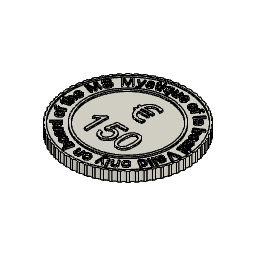
birthday_chip (Autodesk Fusion 360 design; units mm, degrees)
Autodesk Fusion 360 part; units mm, degrees
(part 1 of 2)
sketch "Skizze1" plane through (0, 0, 0) normal (0, 0, 1) x (1, 0, 0)
  circle A0 centre (0, 0) radius 25
  circle A1 centre (0, 0) radius 23.6538
  dimension "d1" = 50
  dimension "d4" = -1.3462
  constraint coincident A0.centre A1.centre
  measures "d1" diameter of A0
extrude "Extrusion1" add sketch "Skizze1" along normal blind 4 contours A0 | A1
sketch "Skizze2" plane through (0, 0, 4) normal (0, 0, 1) x (-1, 0, 0)
  circle A0 centre (0, 0) radius 25
  circle A1 centre (0, 0) radius 24.1386
  dimension "d5" = -0.8614
extrude "Extrusion2" cut sketch "Skizze2" against normal blind 0.6 contours A1
sketch "Skizze3" plane through (0, 0, 3.4) normal (0, 0, 1) x (-1, 0, 0)
  circle A0 centre (0, 0) radius 24.1386
  circle A1 centre (0, 0) radius 17.6628
  circle A2 centre (0, 0) radius 16.7912
  dimension "d8" = -6.4758
  dimension "d9" = -7.3474
extrude "Extrusion3" add sketch "Skizze3" along normal blind 0.6 contours A1
sketch "Skizze4" plane through (0, 0, 3.4) normal (0, 0, 1) x (-1, 0, 0)
  circle A0 centre (0, 0) radius 16.7912
  spline S0 degree 2 poles (-0.7975, -6.5191) (-0.2245, -6.5191) (0.1643, -6.2428) knots 0 0 0 1 1 1
  spline S1 degree 2 poles (0.1643, -6.2428) (0.3962, -6.0791) (0.5838, -5.779) knots 0 0 0 1 1 1
  spline S2 degree 2 poles (0.5838, -5.779) (0.7748, -5.4686) (0.8089, -5.1889) knots 0 0 0 1 1 1
  line L0 (0.8089, -5.1889) -> (-1.5172, -5.1889)
  line L1 (-1.5172, -5.1889) -> (-1.4251, -4.7319)
  line L2 (-1.4251, -4.7319) -> (0.8634, -4.7319)
  spline S3 degree 2 poles (0.8634, -4.7319) (0.8669, -4.6603) (0.8669, -4.5955) knots 0 0 0 1 1 1
  spline S4 degree 2 poles (0.8669, -4.5955) (0.8669, -4.3329) (0.8634, -4.2817) knots 0 0 0 1 1 1
  line L3 (0.8634, -4.2817) -> (-1.333, -4.2817)
  line L4 (-1.333, -4.2817) -> (-1.2375, -3.8247)
  line L5 (-1.2375, -3.8247) -> (0.7918, -3.8247)
  spline S5 degree 2 poles (0.7918, -3.8247) (0.6486, -3.0437) (0.1029, -2.7162) knots 0 0 0 1 1 1
  spline S6 degree 2 poles (0.1029, -2.7162) (-0.2894, -2.4809) (-0.7464, -2.4809) knots 0 0 0 1 1 1
  spline S7 degree 2 poles (-0.7464, -2.4809) (-1.3842, -2.4809) (-1.7423, -2.8151) knots 0 0 0 1 1 1
  line L6 (-1.7423, -2.8151) -> (-1.7423, -2.1126)
  spline S8 degree 2 poles (-1.7423, -2.1126) (-1.316, -1.9147) (-0.8009, -1.9147) knots 0 0 0 1 1 1
  spline S9 degree 2 poles (-0.8009, -1.9147) (0.7407, -1.9147) (1.283, -3.1971) knots 0 0 0 1 1 1
  spline S10 degree 2 poles (1.283, -3.1971) (1.3921, -3.4563) (1.4705, -3.8247) knots 0 0 0 1 1 1
  line L7 (1.4705, -3.8247) -> (1.9924, -3.8247)
  line L8 (1.9924, -3.8247) -> (1.8969, -4.2817)
  line L9 (1.8969, -4.2817) -> (1.5388, -4.2817)
  spline S11 degree 2 poles (1.5388, -4.2817) (1.549, -4.425) (1.549, -4.5921) knots 0 0 0 1 1 1
  spline S12 degree 2 poles (1.549, -4.5921) (1.549, -4.6603) (1.5456, -4.7319) knots 0 0 0 1 1 1
  line L10 (1.5456, -4.7319) -> (1.9924, -4.7319)
  line L11 (1.9924, -4.7319) -> (1.8969, -5.1889)
  line L12 (1.8969, -5.1889) -> (1.5012, -5.1889)
  spline S13 degree 2 poles (1.5012, -5.1889) (1.2898, -6.3008) (0.3996, -6.7851) knots 0 0 0 1 1 1
  spline S14 degree 2 poles (0.3996, -6.7851) (-0.1495, -7.0853) (-0.8112, -7.0853) knots 0 0 0 1 1 1
  spline S15 degree 2 poles (-0.8112, -7.0853) (-1.4456, -7.0853) (-1.8787, -6.809) knots 0 0 0 1 1 1
  line L13 (-1.8787, -6.809) -> (-1.7423, -6.1746)
  spline S16 degree 2 poles (-1.7423, -6.1746) (-1.3262, -6.5191) (-0.7975, -6.5191) knots 0 0 0 1 1 1
  line L14 (3.1793, 5.8035) -> (3.7932, 5.8035)
  line L15 (3.7932, 5.8035) -> (3.7932, 1.8915)
  spline S17 degree 2 poles (3.7932, 1.8915) (4.0149, 2.103) (4.3747, 2.3145) knots 0 0 0 1 1 1
  spline S18 degree 2 poles (4.3747, 2.3145) (4.7345, 2.5259) (5.021, 2.6316) knots 0 0 0 1 1 1
  line L16 (5.021, 2.6316) -> (5.021, 2.0382)
  spline S19 degree 2 poles (5.021, 2.0382) (4.506, 1.796) (4.1206, 1.4516) knots 0 0 0 1 1 1
  spline S20 degree 2 poles (4.1206, 1.4516) (3.7352, 1.1071) (3.5749, 0.7831) knots 0 0 0 1 1 1
  line L17 (3.5749, 0.7831) -> (3.1793, 0.7831)
  line L18 (3.1793, 0.7831) -> (3.1793, 5.8035)
  line L19 (1.607, 4.4939) -> (0.9624, 4.4393)
  spline S21 degree 2 poles (0.9624, 4.4393) (0.8907, 4.91) (0.6298, 5.147) knots 0 0 0 1 1 1
  spline S22 degree 2 poles (0.6298, 5.147) (0.3689, 5.384) (0.0006, 5.384) knots 0 0 0 1 1 1
  spline S23 degree 2 poles (0.0006, 5.384) (-0.4428, 5.384) (-0.7498, 5.0498) knots 0 0 0 1 1 1
  spline S24 degree 2 poles (-0.7498, 5.0498) (-1.0567, 4.7156) (-1.0567, 4.163) knots 0 0 0 1 1 1
  spline S25 degree 2 poles (-1.0567, 4.163) (-1.0567, 3.6378) (-0.7617, 3.3342) knots 0 0 0 1 1 1
  spline S26 degree 2 poles (-0.7617, 3.3342) (-0.4667, 3.0307) (0.0108, 3.0307) knots 0 0 0 1 1 1
  spline S27 degree 2 poles (0.0108, 3.0307) (0.3075, 3.0307) (0.5463, 3.1654) knots 0 0 0 1 1 1
  spline S28 degree 2 poles (0.5463, 3.1654) (0.785, 3.3001) (0.9214, 3.515) knots 0 0 0 1 1 1
  line L20 (0.9214, 3.515) -> (1.4978, 3.44)
  line L21 (1.4978, 3.44) -> (1.0135, 0.8718)
  line L22 (1.0135, 0.8718) -> (-1.4728, 0.8718)
  line L23 (-1.4728, 0.8718) -> (-1.4728, 1.4584)
  line L24 (-1.4728, 1.4584) -> (0.5224, 1.4584)
  line L25 (0.5224, 1.4584) -> (0.7918, 2.8022)
  spline S29 degree 2 poles (0.7918, 2.8022) (0.3416, 2.4884) (-0.1529, 2.4884) knots 0 0 0 1 1 1
  spline S30 degree 2 poles (-0.1529, 2.4884) (-0.8078, 2.4884) (-1.258, 2.942) knots 0 0 0 1 1 1
  spline S31 degree 2 poles (-1.258, 2.942) (-1.7082, 3.3956) (-1.7082, 4.1085) knots 0 0 0 1 1 1
  spline S32 degree 2 poles (-1.7082, 4.1085) (-1.7082, 4.7872) (-1.3125, 5.2817) knots 0 0 0 1 1 1
  spline S33 degree 2 poles (-1.3125, 5.2817) (-0.8316, 5.8888) (0.0006, 5.8888) knots 0 0 0 1 1 1
  spline S34 degree 2 poles (0.0006, 5.8888) (0.6827, 5.8888) (1.1141, 5.5068) knots 0 0 0 1 1 1
  spline S35 degree 2 poles (1.1141, 5.5068) (1.5456, 5.1248) (1.607, 4.4939) knots 0 0 0 1 1 1
  spline S36 degree 2 poles (-2.2778, 3.3377) (-2.2778, 2.4509) (-2.4602, 1.9103) knots 0 0 0 1 1 1
  spline S37 degree 2 poles (-2.4602, 1.9103) (-2.6427, 1.3697) (-3.0025, 1.0764) knots 0 0 0 1 1 1
  spline S38 degree 2 poles (-3.0025, 1.0764) (-3.3623, 0.7831) (-3.908, 0.7831) knots 0 0 0 1 1 1
  spline S39 degree 2 poles (-3.908, 0.7831) (-4.3105, 0.7831) (-4.614, 0.9451) knots 0 0 0 1 1 1
  spline S40 degree 2 poles (-4.614, 0.9451) (-4.9176, 1.1071) (-5.1154, 1.4123) knots 0 0 0 1 1 1
  spline S41 degree 2 poles (-5.1154, 1.4123) (-5.3132, 1.7176) (-5.4258, 2.1559) knots 0 0 0 1 1 1
  spline S42 degree 2 poles (-5.4258, 2.1559) (-5.5383, 2.5941) (-5.5383, 3.3377) knots 0 0 0 1 1 1
  spline S43 degree 2 poles (-5.5383, 3.3377) (-5.5383, 4.2176) (-5.3576, 4.7582) knots 0 0 0 1 1 1
  spline S44 degree 2 poles (-5.3576, 4.7582) (-5.1768, 5.2988) (-4.817, 5.5938) knots 0 0 0 1 1 1
  spline S45 degree 2 poles (-4.817, 5.5938) (-4.4572, 5.8888) (-3.908, 5.8888) knots 0 0 0 1 1 1
  spline S46 degree 2 poles (-3.908, 5.8888) (-3.185, 5.8888) (-2.7723, 5.3704) knots 0 0 0 1 1 1
  spline S47 degree 2 poles (-2.7723, 5.3704) (-2.2778, 4.7462) (-2.2778, 3.3377) knots 0 0 0 1 1 1
  spline S48 degree 2 poles (-2.9087, 3.3377) (-2.9087, 4.5689) (-3.1969, 4.9765) knots 0 0 0 1 1 1
  spline S49 degree 2 poles (-3.1969, 4.9765) (-3.4851, 5.384) (-3.908, 5.384) knots 0 0 0 1 1 1
  spline S50 degree 2 poles (-3.908, 5.384) (-4.331, 5.384) (-4.6192, 4.9748) knots 0 0 0 1 1 1
  spline S51 degree 2 poles (-4.6192, 4.9748) (-4.9074, 4.5655) (-4.9074, 3.3377) knots 0 0 0 1 1 1
  spline S52 degree 2 poles (-4.9074, 3.3377) (-4.9074, 2.103) (-4.6192, 1.6971) knots 0 0 0 1 1 1
  spline S53 degree 2 poles (-4.6192, 1.6971) (-4.331, 1.2913) (-3.9012, 1.2913) knots 0 0 0 1 1 1
  spline S54 degree 2 poles (-3.9012, 1.2913) (-3.4783, 1.2913) (-3.2259, 1.6494) knots 0 0 0 1 1 1
  spline S55 degree 2 poles (-3.2259, 1.6494) (-2.9087, 2.1064) (-2.9087, 3.3377) knots 0 0 0 1 1 1
sketch "Skizze5" plane through (0, 0, 3.4) normal (0, 0, 1) x (-1, 0, 0)
  circle A0 centre (0, 0) radius 16.7912
  spline S0 degree 2 poles (-0.97, -11.1344) (0.0614, -11.1344) (0.7613, -10.6371) knots 0 0 0 1 1 1
  spline S1 degree 2 poles (0.7613, -10.6371) (1.1787, -10.3424) (1.5164, -9.8022) knots 0 0 0 1 1 1
  spline S2 degree 2 poles (1.5164, -9.8022) (1.8602, -9.2435) (1.9216, -8.7401) knots 0 0 0 1 1 1
  line L0 (1.9216, -8.7401) -> (-2.2653, -8.7401)
  line L1 (-2.2653, -8.7401) -> (-2.0996, -7.9175)
  line L2 (-2.0996, -7.9175) -> (2.0198, -7.9175)
  spline S3 degree 2 poles (2.0198, -7.9175) (2.0259, -7.7885) (2.0259, -7.6719) knots 0 0 0 1 1 1
  spline S4 degree 2 poles (2.0259, -7.6719) (2.0259, -7.1992) (2.0198, -7.1071) knots 0 0 0 1 1 1
  line L3 (2.0198, -7.1071) -> (-1.9338, -7.1071)
  line L4 (-1.9338, -7.1071) -> (-1.7619, -6.2844)
  line L5 (-1.7619, -6.2844) -> (1.8909, -6.2844)
  spline S5 degree 2 poles (1.8909, -6.2844) (1.633, -4.8786) (0.6508, -4.2892) knots 0 0 0 1 1 1
  spline S6 degree 2 poles (0.6508, -4.2892) (-0.0553, -3.8656) (-0.8779, -3.8656) knots 0 0 0 1 1 1
  spline S7 degree 2 poles (-0.8779, -3.8656) (-2.0259, -3.8656) (-2.6705, -4.4673) knots 0 0 0 1 1 1
  line L6 (-2.6705, -4.4673) -> (-2.6705, -3.2026)
  spline S8 degree 2 poles (-2.6705, -3.2026) (-1.9031, -2.8465) (-0.9761, -2.8465) knots 0 0 0 1 1 1
  spline S9 degree 2 poles (-0.9761, -2.8465) (1.7988, -2.8465) (2.7749, -5.1548) knots 0 0 0 1 1 1
  spline S10 degree 2 poles (2.7749, -5.1548) (2.9714, -5.6214) (3.1126, -6.2844) knots 0 0 0 1 1 1
  line L7 (3.1126, -6.2844) -> (4.0518, -6.2844)
  line L8 (4.0518, -6.2844) -> (3.8799, -7.1071)
  line L9 (3.8799, -7.1071) -> (3.2353, -7.1071)
  spline S11 degree 2 poles (3.2353, -7.1071) (3.2538, -7.3649) (3.2538, -7.6658) knots 0 0 0 1 1 1
  spline S12 degree 2 poles (3.2538, -7.6658) (3.2538, -7.7885) (3.2476, -7.9175) knots 0 0 0 1 1 1
  line L10 (3.2476, -7.9175) -> (4.0518, -7.9175)
  line L11 (4.0518, -7.9175) -> (3.8799, -8.7401)
  line L12 (3.8799, -8.7401) -> (3.1678, -8.7401)
  spline S13 degree 2 poles (3.1678, -8.7401) (2.7872, -10.7415) (1.1849, -11.6132) knots 0 0 0 1 1 1
  spline S14 degree 2 poles (1.1849, -11.6132) (0.1965, -12.1535) (-0.9945, -12.1535) knots 0 0 0 1 1 1
  spline S15 degree 2 poles (-0.9945, -12.1535) (-2.1364, -12.1535) (-2.9161, -11.6562) knots 0 0 0 1 1 1
  line L13 (-2.9161, -11.6562) -> (-2.6705, -10.5143)
  spline S16 degree 2 poles (-2.6705, -10.5143) (-1.9216, -11.1344) (-0.97, -11.1344) knots 0 0 0 1 1 1
  line L14 (6.1883, 11.0464) -> (7.2933, 11.0464)
  line L15 (7.2933, 11.0464) -> (7.2933, 4.0048)
  spline S17 degree 2 poles (7.2933, 4.0048) (7.6924, 4.3854) (8.34, 4.766) knots 0 0 0 1 1 1
  spline S18 degree 2 poles (8.34, 4.766) (8.9877, 5.1467) (9.5034, 5.337) knots 0 0 0 1 1 1
  line L16 (9.5034, 5.337) -> (9.5034, 4.2688)
  spline S19 degree 2 poles (9.5034, 4.2688) (8.5764, 3.8329) (7.8827, 3.2128) knots 0 0 0 1 1 1
  spline S20 degree 2 poles (7.8827, 3.2128) (7.1889, 2.5928) (6.9004, 2.0096) knots 0 0 0 1 1 1
  line L17 (6.9004, 2.0096) -> (6.1883, 2.0096)
  line L18 (6.1883, 2.0096) -> (6.1883, 11.0464)
  line L19 (3.3581, 8.6889) -> (2.1978, 8.5907)
  spline S21 degree 2 poles (2.1978, 8.5907) (2.0689, 9.4379) (1.5992, 9.8646) knots 0 0 0 1 1 1
  spline S22 degree 2 poles (1.5992, 9.8646) (1.1296, 10.2913) (0.4666, 10.2913) knots 0 0 0 1 1 1
  spline S23 degree 2 poles (0.4666, 10.2913) (-0.3315, 10.2913) (-0.884, 9.6896) knots 0 0 0 1 1 1
  spline S24 degree 2 poles (-0.884, 9.6896) (-1.4366, 9.088) (-1.4366, 8.0935) knots 0 0 0 1 1 1
  spline S25 degree 2 poles (-1.4366, 8.0935) (-1.4366, 7.148) (-0.9055, 6.6016) knots 0 0 0 1 1 1
  spline S26 degree 2 poles (-0.9055, 6.6016) (-0.3745, 6.0553) (0.485, 6.0553) knots 0 0 0 1 1 1
  spline S27 degree 2 poles (0.485, 6.0553) (1.0191, 6.0553) (1.4488, 6.2977) knots 0 0 0 1 1 1
  spline S28 degree 2 poles (1.4488, 6.2977) (1.8786, 6.5402) (2.1241, 6.927) knots 0 0 0 1 1 1
  line L20 (2.1241, 6.927) -> (3.1617, 6.792)
  line L21 (3.1617, 6.792) -> (2.2899, 2.1692)
  line L22 (2.2899, 2.1692) -> (-2.1855, 2.1692)
  line L23 (-2.1855, 2.1692) -> (-2.1855, 3.2251)
  line L24 (-2.1855, 3.2251) -> (1.4059, 3.2251)
  line L25 (1.4059, 3.2251) -> (1.8909, 5.6439)
  spline S29 degree 2 poles (1.8909, 5.6439) (1.0805, 5.0791) (0.1903, 5.0791) knots 0 0 0 1 1 1
  spline S30 degree 2 poles (0.1903, 5.0791) (-0.9884, 5.0791) (-1.7988, 5.8956) knots 0 0 0 1 1 1
  spline S31 degree 2 poles (-1.7988, 5.8956) (-2.6091, 6.7121) (-2.6091, 7.9952) knots 0 0 0 1 1 1
  spline S32 degree 2 poles (-2.6091, 7.9952) (-2.6091, 9.2169) (-1.897, 10.1071) knots 0 0 0 1 1 1
  spline S33 degree 2 poles (-1.897, 10.1071) (-1.0314, 11.1999) (0.4666, 11.1999) knots 0 0 0 1 1 1
  spline S34 degree 2 poles (0.4666, 11.1999) (1.6944, 11.1999) (2.471, 10.5123) knots 0 0 0 1 1 1
  spline S35 degree 2 poles (2.471, 10.5123) (3.2476, 9.8247) (3.3581, 8.6889) knots 0 0 0 1 1 1
  spline S36 degree 2 poles (-3.6344, 6.6078) (-3.6344, 5.0116) (-3.9628, 4.0385) knots 0 0 0 1 1 1
  spline S37 degree 2 poles (-3.9628, 4.0385) (-4.2913, 3.0655) (-4.9389, 2.5375) knots 0 0 0 1 1 1
  spline S38 degree 2 poles (-4.9389, 2.5375) (-5.5866, 2.0096) (-6.5689, 2.0096) knots 0 0 0 1 1 1
  spline S39 degree 2 poles (-6.5689, 2.0096) (-7.2933, 2.0096) (-7.8397, 2.3012) knots 0 0 0 1 1 1
  spline S40 degree 2 poles (-7.8397, 2.3012) (-8.3861, 2.5928) (-8.7422, 3.1422) knots 0 0 0 1 1 1
  spline S41 degree 2 poles (-8.7422, 3.1422) (-9.0982, 3.6917) (-9.3008, 4.4806) knots 0 0 0 1 1 1
  spline S42 degree 2 poles (-9.3008, 4.4806) (-9.5034, 5.2694) (-9.5034, 6.6078) knots 0 0 0 1 1 1
  spline S43 degree 2 poles (-9.5034, 6.6078) (-9.5034, 8.1917) (-9.178, 9.1647) knots 0 0 0 1 1 1
  spline S44 degree 2 poles (-9.178, 9.1647) (-8.8527, 10.1378) (-8.205, 10.6688) knots 0 0 0 1 1 1
  spline S45 degree 2 poles (-8.205, 10.6688) (-7.5573, 11.1999) (-6.5689, 11.1999) knots 0 0 0 1 1 1
  spline S46 degree 2 poles (-6.5689, 11.1999) (-5.2674, 11.1999) (-4.5246, 10.2667) knots 0 0 0 1 1 1
  spline S47 degree 2 poles (-4.5246, 10.2667) (-3.6344, 9.1432) (-3.6344, 6.6078) knots 0 0 0 1 1 1
  spline S48 degree 2 poles (-4.7701, 6.6078) (-4.7701, 8.824) (-5.2889, 9.5576) knots 0 0 0 1 1 1
  spline S49 degree 2 poles (-5.2889, 9.5576) (-5.8076, 10.2913) (-6.5689, 10.2913) knots 0 0 0 1 1 1
  spline S50 degree 2 poles (-6.5689, 10.2913) (-7.3301, 10.2913) (-7.8489, 9.5546) knots 0 0 0 1 1 1
  spline S51 degree 2 poles (-7.8489, 9.5546) (-8.3677, 8.8179) (-8.3677, 6.6078) knots 0 0 0 1 1 1
  spline S52 degree 2 poles (-8.3677, 6.6078) (-8.3677, 4.3854) (-7.8489, 3.6548) knots 0 0 0 1 1 1
  spline S53 degree 2 poles (-7.8489, 3.6548) (-7.3301, 2.9243) (-6.5566, 2.9243) knots 0 0 0 1 1 1
  spline S54 degree 2 poles (-6.5566, 2.9243) (-5.7954, 2.9243) (-5.3411, 3.5689) knots 0 0 0 1 1 1
  spline S55 degree 2 poles (-5.3411, 3.5689) (-4.7701, 4.3915) (-4.7701, 6.6078) knots 0 0 0 1 1 1
extrude "Extrusion5" add sketch "Skizze5" along normal blind 0.6 contours S0 S1 S2 L0 L1 L2 S3 S4 L3 L4 L5 S5 S6 S7 L6 S8 S9 S10 L7 L8 L9 S11 S12 L10 L11 L12 S13 S14 S15 L13 S16 | L14 L15 S17 S18 L16 S19 S20 L17 L18 | L19 S21 S22 S23 S24 S25 S26 S27 S28 L20 L21 L22 L23 L24 L25 S29 S30 S31 S32 S33 S34 S35 | S36 S37 S38 S39 S40 S41 S42 S43 S44 S45 S46 S47
sketch "Skizze7" plane through (0, 0, 4) normal (0, 0, 1) x (-1, 0, 0)
  circle A0 centre (0, 0) radius 24.1386
  circle A1 centre (0, 0) radius 25
  circle A2 centre (0, -26) radius 1.329
  circle A3 centre (2.7177, -25.8576) radius 1.329
  circle A4 centre (5.4057, -25.4318) radius 1.329
  circle A5 centre (8.0344, -24.7275) radius 1.329
  circle A6 centre (10.5752, -23.7522) radius 1.329
  circle A7 centre (13, -22.5167) radius 1.329
  circle A8 centre (15.2824, -21.0344) radius 1.329
  circle A9 centre (17.3974, -19.3218) radius 1.329
  circle A10 centre (19.3218, -17.3974) radius 1.329
  circle A11 centre (21.0344, -15.2824) radius 1.329
  circle A12 centre (22.5167, -13) radius 1.329
  circle A13 centre (23.7522, -10.5752) radius 1.329
  circle A14 centre (24.7275, -8.0344) radius 1.329
  circle A15 centre (25.4318, -5.4057) radius 1.329
  circle A16 centre (25.8576, -2.7177) radius 1.329
  circle A17 centre (26, 0) radius 1.329
  circle A18 centre (25.8576, 2.7177) radius 1.329
  circle A19 centre (25.4318, 5.4057) radius 1.329
  circle A20 centre (24.7275, 8.0344) radius 1.329
  circle A21 centre (23.7522, 10.5752) radius 1.329
  circle A22 centre (22.5167, 13) radius 1.329
  circle A23 centre (21.0344, 15.2824) radius 1.329
  circle A24 centre (19.3218, 17.3974) radius 1.329
  circle A25 centre (17.3974, 19.3218) radius 1.329
  circle A26 centre (15.2824, 21.0344) radius 1.329
  circle A27 centre (13, 22.5167) radius 1.329
  circle A28 centre (10.5752, 23.7522) radius 1.329
  circle A29 centre (8.0344, 24.7275) radius 1.329
  circle A30 centre (5.4057, 25.4318) radius 1.329
  circle A31 centre (2.7177, 25.8576) radius 1.329
  circle A32 centre (0, 26) radius 1.329
  circle A33 centre (-2.7177, 25.8576) radius 1.329
  circle A34 centre (-5.4057, 25.4318) radius 1.329
  circle A35 centre (-8.0344, 24.7275) radius 1.329
  circle A36 centre (-10.5752, 23.7522) radius 1.329
  circle A37 centre (-13, 22.5167) radius 1.329
  circle A38 centre (-15.2824, 21.0344) radius 1.329
  circle A39 centre (-17.3974, 19.3218) radius 1.329
  circle A40 centre (-19.3218, 17.3974) radius 1.329
  circle A41 centre (-21.0344, 15.2824) radius 1.329
  circle A42 centre (-22.5167, 13) radius 1.329
  circle A43 centre (-23.7522, 10.5752) radius 1.329
  circle A44 centre (-24.7275, 8.0344) radius 1.329
  circle A45 centre (-25.4318, 5.4057) radius 1.329
  circle A46 centre (-25.8576, 2.7177) radius 1.329
  circle A47 centre (-26, 0) radius 1.329
  circle A48 centre (-25.8576, -2.7177) radius 1.329
  circle A49 centre (-25.4318, -5.4057) radius 1.329
  circle A50 centre (-24.7275, -8.0344) radius 1.329
  circle A51 centre (-23.7522, -10.5752) radius 1.329
  circle A52 centre (-22.5167, -13) radius 1.329
  circle A53 centre (-21.0344, -15.2824) radius 1.329
  circle A54 centre (-19.3218, -17.3974) radius 1.329
  circle A55 centre (-17.3974, -19.3218) radius 1.329
  circle A56 centre (-15.2824, -21.0344) radius 1.329
  circle A57 centre (-13, -22.5167) radius 1.329
  circle A58 centre (-10.5752, -23.7522) radius 1.329
  circle A59 centre (-8.0344, -24.7275) radius 1.329
  circle A60 centre (-5.4057, -25.4318) radius 1.329
  circle A61 centre (-2.7177, -25.8576) radius 1.329
  dimension "d22" = 2.6579
  dimension "d24" = 360
  measures "d22" diameter of A2
extrude "Extrusion7" cut sketch "Skizze7" against normal blind 10 contours A1 A17 | A1 A18 | A1 A16 | A1 A19 | A1 A15 | A1 A20 | A1 A14 | A1 A21 | A1 A13 | A1 A22 | A1 A12 | A1 A23 | A1 A11 | A1 A24 | A1 A10 | A1 A25 | A1 A9 | A1 A26 | A1 A8 | A1 A27 | A1 A7 | A1 A28 | A1 A6 | A1 A29 | A1 A5 | A1 A30 | A1 A4 | A1 A31 | A1 A3 | A1 A32 | A1 A2 | A1 A33 | A1 A61 | A1 A34 | A1 A60 | A1 A35 | A1 A59 | A1 A36 | A1 A58 | A1 A37 | A1 A57 | A1 A38 | A1 A56 | A1 A39 | A1 A55 | A1 A40 | A1 A54 | A1 A41 | A1 A53 | A1 A42 | A1 A52 | A1 A43 | A1 A51 | A1 A44 | A1 A50 | A1 A45 | A1 A49 | A1 A46 | A1 A48 | A1 A47 picked at (24.8942, -0.1574) picked at (24.7529, 2.6016) picked at (24.7529, -2.6016) picked at (24.3454, 5.1748) picked at (24.3454, -5.1748) picked at (23.6711, 7.6912) picked at (23.6711, -7.6912) picked at (22.7375, 10.1234) picked at (22.7375, -10.1234) picked at (21.5547, 12.4446) picked at (21.5547, -12.4446) picked at (20.1358, 14.6295) picked at (20.1358, -14.6295) picked at (18.4963, 16.6542) picked at (18.4963, -16.6542) picked at (16.6542, 18.4963) picked at (16.6542, -18.4963) picked at (14.6295, 20.1358) picked at (14.6295, -20.1358) picked at (12.4446, 21.5547) picked at (12.4446, -21.5547) picked at (10.1234, 22.7375) picked at (10.1234, -22.7375) picked at (7.6912, 23.6711) picked at (7.6912, -23.6711) picked at (5.1748, 24.3454) picked at (5.1748, -24.3454) picked at (2.6016, 24.7529) picked at (2.6016, -24.7529) picked at (0, 24.8893) picked at (0, -24.8893) picked at (-2.6016, 24.7529) picked at (-2.6016, -24.7529) picked at (-5.1748, 24.3454) picked at (-5.1748, -24.3454) picked at (-7.6912, 23.6711) picked at (-7.6912, -23.6711) picked at (-10.1234, 22.7375) picked at (-10.1234, -22.7375) picked at (-12.4446, 21.5547) picked at (-12.4446, -21.5547) picked at (-14.6295, 20.1358) picked at (-14.6295, -20.1358) picked at (-16.6542, 18.4963) picked at (-16.6542, -18.4963) picked at (-18.4963, 16.6542) picked at (-18.4963, -16.6542) picked at (-20.1264, 14.643) picked at (-20.1264, -14.643) picked at (-21.5595, 12.4366) picked at (-21.5595, -12.4366) picked at (-22.7377, 10.1228) picked at (-22.7377, -10.1228) picked at (-23.6679, 7.7013) picked at (-23.6679, -7.7013) picked at (-24.3506, 5.1528) picked at (-24.3506, -5.1528) picked at (-24.7545, 2.5886) picked at (-24.7545, -2.5886) picked at (-24.8893, 0)
sketch "Skizze8" plane through (0, 0, 3.4) normal (0, 0, 1) x (-1, 0, 0)
  circle A0 centre (0, 0) radius 24.1386
  circle A1 centre (0, 0) radius 17.6628
  circle A2 centre (0, 0) radius 19.3942
  line L0 (-19.2805, 2.1162) -> (-23.3373, 1.0985)
  line L1 (-23.3373, 1.0985) -> (-23.2683, 1.6529)
  line L2 (-23.2683, 1.6529) -> (-20.3315, 2.3087)
  spline S0 degree 2 poles (-20.3315, 2.3087) (-19.9785, 2.3881) (-19.6727, 2.4331) knots 0 0 0 1 1 1
  spline S1 degree 2 poles (-19.6727, 2.4331) (-19.9783, 2.5623) (-20.2803, 2.7205) knots 0 0 0 1 1 1
  line L3 (-20.2803, 2.7205) -> (-22.9616, 4.116)
  line L4 (-22.9616, 4.116) -> (-22.8966, 4.6387)
  line L5 (-22.8966, 4.6387) -> (-19.2151, 2.6415)
  line L6 (-19.2151, 2.6415) -> (-19.2805, 2.1162)
  spline S2 degree 2 poles (-18.6857, 6.4104) (-18.5469, 6.09) (-18.5295, 5.8275) knots 0 0 0 1 1 1
  spline S3 degree 2 poles (-18.5295, 5.8275) (-18.5122, 5.565) (-18.5943, 5.2952) knots 0 0 0 1 1 1
  spline S4 degree 2 poles (-18.5943, 5.2952) (-18.73, 4.8499) (-19.0204, 4.6769) knots 0 0 0 1 1 1
  spline S5 degree 2 poles (-19.0204, 4.6769) (-19.3109, 4.504) (-19.6493, 4.6071) knots 0 0 0 1 1 1
  spline S6 degree 2 poles (-19.6493, 4.6071) (-19.8478, 4.6675) (-19.9845, 4.8079) knots 0 0 0 1 1 1
  spline S7 degree 2 poles (-19.9845, 4.8079) (-20.1211, 4.9482) (-20.1758, 5.1248) knots 0 0 0 1 1 1
  spline S8 degree 2 poles (-20.1758, 5.1248) (-20.2304, 5.3013) (-20.2255, 5.5001) knots 0 0 0 1 1 1
  spline S9 degree 2 poles (-20.2255, 5.5001) (-20.2201, 5.6458) (-20.1702, 5.9282) knots 0 0 0 1 1 1
  spline S10 degree 2 poles (-20.1702, 5.9282) (-20.0674, 6.5031) (-20.0792, 6.7931) knots 0 0 0 1 1 1
  spline S11 degree 2 poles (-20.0792, 6.7931) (-20.1726, 6.8244) (-20.198, 6.8321) knots 0 0 0 1 1 1
  spline S12 degree 2 poles (-20.198, 6.8321) (-20.4779, 6.9174) (-20.632, 6.8225) knots 0 0 0 1 1 1
  spline S13 degree 2 poles (-20.632, 6.8225) (-20.8407, 6.6942) (-20.9461, 6.3481) knots 0 0 0 1 1 1
  spline S14 degree 2 poles (-20.9461, 6.3481) (-21.0446, 6.0249) (-20.9782, 5.8364) knots 0 0 0 1 1 1
  spline S15 degree 2 poles (-20.9782, 5.8364) (-20.9119, 5.6479) (-20.6468, 5.4866) knots 0 0 0 1 1 1
  line L7 (-20.6468, 5.4866) -> (-20.8443, 5.0573)
  spline S16 degree 2 poles (-20.8443, 5.0573) (-21.1133, 5.2059) (-21.2475, 5.3998) knots 0 0 0 1 1 1
  spline S17 degree 2 poles (-21.2475, 5.3998) (-21.3817, 5.5936) (-21.3965, 5.8873) knots 0 0 0 1 1 1
  spline S18 degree 2 poles (-21.3965, 5.8873) (-21.4114, 6.1811) (-21.3052, 6.5297) knots 0 0 0 1 1 1
  spline S19 degree 2 poles (-21.3052, 6.5297) (-21.1998, 6.8758) (-21.0524, 7.0673) knots 0 0 0 1 1 1
  spline S20 degree 2 poles (-21.0524, 7.0673) (-20.9051, 7.2588) (-20.7507, 7.323) knots 0 0 0 1 1 1
  spline S21 degree 2 poles (-20.7507, 7.323) (-20.5962, 7.3872) (-20.3955, 7.3706) knots 0 0 0 1 1 1
  spline S22 degree 2 poles (-20.3955, 7.3706) (-20.2715, 7.3579) (-19.9661, 7.2648) knots 0 0 0 1 1 1
  line L8 (-19.9661, 7.2648) -> (-19.3553, 7.0788)
  spline S23 degree 2 poles (-19.3553, 7.0788) (-18.7166, 6.8842) (-18.5384, 6.862) knots 0 0 0 1 1 1
  spline S24 degree 2 poles (-18.5384, 6.862) (-18.3603, 6.8397) (-18.1787, 6.8789) knots 0 0 0 1 1 1
  line L9 (-18.1787, 6.8789) -> (-18.3244, 6.4005)
  spline S25 degree 2 poles (-18.3244, 6.4005) (-18.4886, 6.3726) (-18.6857, 6.4104) knots 0 0 0 1 1 1
  spline S26 degree 2 poles (-19.7204, 6.6838) (-19.6945, 6.4034) (-19.7752, 5.8829) knots 0 0 0 1 1 1
  spline S27 degree 2 poles (-19.7752, 5.8829) (-19.8205, 5.5881) (-19.8053, 5.4555) knots 0 0 0 1 1 1
  spline S28 degree 2 poles (-19.8053, 5.4555) (-19.79, 5.3229) (-19.7114, 5.2295) knots 0 0 0 1 1 1
  spline S29 degree 2 poles (-19.7114, 5.2295) (-19.6328, 5.136) (-19.5132, 5.0996) knots 0 0 0 1 1 1
  spline S30 degree 2 poles (-19.5132, 5.0996) (-19.33, 5.0438) (-19.1656, 5.1452) knots 0 0 0 1 1 1
  spline S31 degree 2 poles (-19.1656, 5.1452) (-19.0012, 5.2467) (-18.9198, 5.5139) knots 0 0 0 1 1 1
  spline S32 degree 2 poles (-18.9198, 5.5139) (-18.8392, 5.7786) (-18.8922, 6.02) knots 0 0 0 1 1 1
  spline S33 degree 2 poles (-18.8922, 6.02) (-18.9452, 6.2614) (-19.1168, 6.4194) knots 0 0 0 1 1 1
  spline S34 degree 2 poles (-19.1168, 6.4194) (-19.2496, 6.5404) (-19.5524, 6.6327) knots 0 0 0 1 1 1
  line L10 (-19.5524, 6.6327) -> (-19.7204, 6.6838)
  line L11 (-17.9265, 7.4055) -> (-21.511, 8.9422)
  line L12 (-21.511, 8.9422) -> (-21.3224, 9.3823)
  line L13 (-21.3224, 9.3823) -> (-17.7378, 7.8457)
  line L14 (-17.7378, 7.8457) -> (-17.9265, 7.4055)
  line L15 (-20.4138, 10.0302) -> (-20.9054, 10.2783)
  line L16 (-20.9054, 10.2783) -> (-20.6897, 10.7058)
  line L17 (-20.6897, 10.7058) -> (-20.198, 10.4577)
  line L18 (-20.198, 10.4577) -> (-20.4138, 10.0302)
  line L19 (-17.4237, 8.5211) -> (-19.9459, 9.7941)
  line L20 (-19.9459, 9.7941) -> (-19.7302, 10.2216)
  line L21 (-19.7302, 10.2216) -> (-17.208, 8.9486)
  line L22 (-17.208, 8.9486) -> (-17.4237, 8.5211)
  line L23 (-15.8881, 11.1429) -> (-16.1869, 11.3372)
  spline S35 degree 2 poles (-16.1869, 11.3372) (-15.9811, 10.8828) (-16.2654, 10.4457) knots 0 0 0 1 1 1
  spline S36 degree 2 poles (-16.2654, 10.4457) (-16.4496, 10.1625) (-16.7602, 10.0266) knots 0 0 0 1 1 1
  spline S37 degree 2 poles (-16.7602, 10.0266) (-17.0708, 9.8906) (-17.4355, 9.9422) knots 0 0 0 1 1 1
  spline S38 degree 2 poles (-17.4355, 9.9422) (-17.8003, 9.9938) (-18.1637, 10.2303) knots 0 0 0 1 1 1
  spline S39 degree 2 poles (-18.1637, 10.2303) (-18.5183, 10.4609) (-18.7302, 10.767) knots 0 0 0 1 1 1
  spline S40 degree 2 poles (-18.7302, 10.767) (-18.9421, 11.073) (-18.9422, 11.4095) knots 0 0 0 1 1 1
  spline S41 degree 2 poles (-18.9422, 11.4095) (-18.9423, 11.746) (-18.7523, 12.0381) knots 0 0 0 1 1 1
  spline S42 degree 2 poles (-18.7523, 12.0381) (-18.613, 12.2522) (-18.4139, 12.3607) knots 0 0 0 1 1 1
  spline S43 degree 2 poles (-18.4139, 12.3607) (-18.2148, 12.4692) (-18.0017, 12.4797) knots 0 0 0 1 1 1
  line L24 (-18.0017, 12.4797) -> (-19.1747, 13.2427)
  line L25 (-19.1747, 13.2427) -> (-18.915, 13.6419)
  line L26 (-18.915, 13.6419) -> (-15.6458, 11.5153)
  line L27 (-15.6458, 11.5153) -> (-15.8881, 11.1429)
  spline S44 degree 2 poles (-17.8954, 10.6428) (-17.4405, 10.3469) (-17.0905, 10.3922) knots 0 0 0 1 1 1
  spline S45 degree 2 poles (-17.0905, 10.3922) (-16.7405, 10.4374) (-16.5708, 10.6983) knots 0 0 0 1 1 1
  spline S46 degree 2 poles (-16.5708, 10.6983) (-16.3996, 10.9615) (-16.4951, 11.2854) knots 0 0 0 1 1 1
  spline S47 degree 2 poles (-16.4951, 11.2854) (-16.5906, 11.6094) (-17.0322, 11.8966) knots 0 0 0 1 1 1
  spline S48 degree 2 poles (-17.0322, 11.8966) (-17.5183, 12.2129) (-17.8676, 12.1735) knots 0 0 0 1 1 1
  spline S49 degree 2 poles (-17.8676, 12.1735) (-18.2169, 12.1341) (-18.3954, 11.8598) knots 0 0 0 1 1 1
  spline S50 degree 2 poles (-18.3954, 11.8598) (-18.5694, 11.5922) (-18.4677, 11.2706) knots 0 0 0 1 1 1
  spline S51 degree 2 poles (-18.4677, 11.2706) (-18.3659, 10.9489) (-17.8954, 10.6428) knots 0 0 0 1 1 1
  spline S52 degree 2 poles (-15.2983, 14.1657) (-15.8388, 14.7347) (-15.7827, 15.3091) knots 0 0 0 1 1 1
  spline S53 degree 2 poles (-15.7827, 15.3091) (-15.7347, 15.7877) (-15.3547, 16.1486) knots 0 0 0 1 1 1
  spline S54 degree 2 poles (-15.3547, 16.1486) (-14.9323, 16.5499) (-14.4013, 16.5278) knots 0 0 0 1 1 1
  spline S55 degree 2 poles (-14.4013, 16.5278) (-13.8703, 16.5058) (-13.4067, 16.0178) knots 0 0 0 1 1 1
  spline S56 degree 2 poles (-13.4067, 16.0178) (-13.0311, 15.6224) (-12.9344, 15.2831) knots 0 0 0 1 1 1
  spline S57 degree 2 poles (-12.9344, 15.2831) (-12.8377, 14.9438) (-12.9452, 14.6032) knots 0 0 0 1 1 1
  spline S58 degree 2 poles (-12.9452, 14.6032) (-13.0528, 14.2625) (-13.3208, 14.0078) knots 0 0 0 1 1 1
  spline S59 degree 2 poles (-13.3208, 14.0078) (-13.7509, 13.5992) (-14.2782, 13.6231) knots 0 0 0 1 1 1
  spline S60 degree 2 poles (-14.2782, 13.6231) (-14.8054, 13.6469) (-15.2983, 14.1657) knots 0 0 0 1 1 1
  spline S61 degree 2 poles (-14.9415, 14.5047) (-14.5677, 14.1113) (-14.21, 14.0786) knots 0 0 0 1 1 1
  spline S62 degree 2 poles (-14.21, 14.0786) (-13.8524, 14.0459) (-13.592, 14.2933) knots 0 0 0 1 1 1
  spline S63 degree 2 poles (-13.592, 14.2933) (-13.3336, 14.5388) (-13.3488, 14.8986) knots 0 0 0 1 1 1
  spline S64 degree 2 poles (-13.3488, 14.8986) (-13.3641, 15.2584) (-13.747, 15.6615) knots 0 0 0 1 1 1
  spline S65 degree 2 poles (-13.747, 15.6615) (-14.108, 16.0414) (-14.4666, 16.0732) knots 0 0 0 1 1 1
  spline S66 degree 2 poles (-14.4666, 16.0732) (-14.8252, 16.105) (-15.0817, 15.8613) knots 0 0 0 1 1 1
  spline S67 degree 2 poles (-15.0817, 15.8613) (-15.3421, 15.6139) (-15.3287, 15.256) knots 0 0 0 1 1 1
  spline S68 degree 2 poles (-15.3287, 15.256) (-15.3153, 14.8982) (-14.9415, 14.5047) knots 0 0 0 1 1 1
  line L28 (-11.9592, 15.3117) -> (-13.5627, 17.6378)
  line L29 (-13.5627, 17.6378) -> (-13.2079, 17.8824)
  line L30 (-13.2079, 17.8824) -> (-12.9799, 17.5517)
  spline S69 degree 2 poles (-12.9799, 17.5517) (-12.9879, 18.1117) (-12.5038, 18.4453) knots 0 0 0 1 1 1
  spline S70 degree 2 poles (-12.5038, 18.4453) (-12.2936, 18.5903) (-12.0651, 18.6363) knots 0 0 0 1 1 1
  spline S71 degree 2 poles (-12.0651, 18.6363) (-11.8367, 18.6823) (-11.6646, 18.62) knots 0 0 0 1 1 1
  spline S72 degree 2 poles (-11.6646, 18.62) (-11.4924, 18.5577) (-11.3411, 18.4132) knots 0 0 0 1 1 1
  spline S73 degree 2 poles (-11.3411, 18.4132) (-11.2437, 18.3188) (-11.055, 18.045) knots 0 0 0 1 1 1
  line L31 (-11.055, 18.045) -> (-10.069, 16.6148)
  line L32 (-10.069, 16.6148) -> (-10.4632, 16.343)
  line L33 (-10.4632, 16.343) -> (-11.4386, 17.7579)
  spline S74 degree 2 poles (-11.4386, 17.7579) (-11.6047, 17.9989) (-11.733, 18.0865) knots 0 0 0 1 1 1
  spline S75 degree 2 poles (-11.733, 18.0865) (-11.8613, 18.1742) (-12.0276, 18.1646) knots 0 0 0 1 1 1
  spline S76 degree 2 poles (-12.0276, 18.1646) (-12.1938, 18.155) (-12.3515, 18.0463) knots 0 0 0 1 1 1
  spline S77 degree 2 poles (-12.3515, 18.0463) (-12.6034, 17.8726) (-12.6761, 17.5867) knots 0 0 0 1 1 1
  spline S78 degree 2 poles (-12.6761, 17.5867) (-12.7487, 17.3007) (-12.4407, 16.8539) knots 0 0 0 1 1 1
  line L34 (-12.4407, 16.8539) -> (-11.565, 15.5835)
  line L35 (-11.565, 15.5835) -> (-11.9592, 15.3117)
  line L36 (-9.4256, 16.9517) -> (-11.2756, 20.385)
  line L37 (-11.2756, 20.385) -> (-10.854, 20.6121)
  line L38 (-10.854, 20.6121) -> (-9.0041, 17.1788)
  line L39 (-9.0041, 17.1788) -> (-9.4256, 16.9517)
  line L40 (-7.9532, 16.52) -> (-8.1744, 16.915)
  spline S79 degree 2 poles (-8.1744, 16.915) (-8.0131, 16.9358) (-7.905, 16.9806) knots 0 0 0 1 1 1
  spline S80 degree 2 poles (-7.905, 16.9806) (-7.7575, 17.0417) (-7.6894, 17.1275) knots 0 0 0 1 1 1
  spline S81 degree 2 poles (-7.6894, 17.1275) (-7.6213, 17.2133) (-7.6014, 17.3252) knots 0 0 0 1 1 1
  spline S82 degree 2 poles (-7.6014, 17.3252) (-7.5871, 17.4089) (-7.6027, 17.7105) knots 0 0 0 1 1 1
  spline S83 degree 2 poles (-7.6027, 17.7105) (-7.6057, 17.7525) (-7.6082, 17.835) knots 0 0 0 1 1 1
  line L41 (-7.6082, 17.835) -> (-9.6821, 20.0396)
  line L42 (-9.6821, 20.0396) -> (-9.2053, 20.2372)
  line L43 (-9.2053, 20.2372) -> (-8.0359, 18.9507)
  spline S84 degree 2 poles (-8.0359, 18.9507) (-7.8111, 18.7069) (-7.5962, 18.4245) knots 0 0 0 1 1 1
  spline S85 degree 2 poles (-7.5962, 18.4245) (-7.6462, 18.7608) (-7.6607, 19.0946) knots 0 0 0 1 1 1
  line L44 (-7.6607, 19.0946) -> (-7.7331, 20.8471)
  line L45 (-7.7331, 20.8471) -> (-7.2907, 21.0304)
  line L46 (-7.2907, 21.0304) -> (-7.1839, 17.9647)
  spline S86 degree 2 poles (-7.1839, 17.9647) (-7.1655, 17.4684) (-7.1867, 17.2695) knots 0 0 0 1 1 1
  spline S87 degree 2 poles (-7.1867, 17.2695) (-7.2141, 17.0019) (-7.3242, 16.8368) knots 0 0 0 1 1 1
  spline S88 degree 2 poles (-7.3242, 16.8368) (-7.4343, 16.6717) (-7.6457, 16.5841) knots 0 0 0 1 1 1
  spline S89 degree 2 poles (-7.6457, 16.5841) (-7.7735, 16.5311) (-7.9532, 16.52) knots 0 0 0 1 1 1
  spline S90 degree 2 poles (-4.7618, 20.2985) (-4.8918, 21.0725) (-4.5241, 21.5173) knots 0 0 0 1 1 1
  spline S91 degree 2 poles (-4.5241, 21.5173) (-4.2166, 21.8872) (-3.6998, 21.974) knots 0 0 0 1 1 1
  spline S92 degree 2 poles (-3.6998, 21.974) (-3.1252, 22.0705) (-2.6973, 21.7553) knots 0 0 0 1 1 1
  spline S93 degree 2 poles (-2.6973, 21.7553) (-2.2694, 21.44) (-2.158, 20.7763) knots 0 0 0 1 1 1
  spline S94 degree 2 poles (-2.158, 20.7763) (-2.0676, 20.2385) (-2.1772, 19.9031) knots 0 0 0 1 1 1
  spline S95 degree 2 poles (-2.1772, 19.9031) (-2.2868, 19.5677) (-2.5664, 19.3454) knots 0 0 0 1 1 1
  spline S96 degree 2 poles (-2.5664, 19.3454) (-2.846, 19.1231) (-3.2107, 19.0619) knots 0 0 0 1 1 1
  spline S97 degree 2 poles (-3.2107, 19.0619) (-3.7958, 18.9636) (-4.2195, 19.2782) knots 0 0 0 1 1 1
  spline S98 degree 2 poles (-4.2195, 19.2782) (-4.6433, 19.5928) (-4.7618, 20.2985) knots 0 0 0 1 1 1
  spline S99 degree 2 poles (-4.2764, 20.38) (-4.1865, 19.8448) (-3.9083, 19.6178) knots 0 0 0 1 1 1
  spline S100 degree 2 poles (-3.9083, 19.6178) (-3.6301, 19.3907) (-3.2759, 19.4502) knots 0 0 0 1 1 1
  spline S101 degree 2 poles (-3.2759, 19.4502) (-2.9244, 19.5092) (-2.7358, 19.816) knots 0 0 0 1 1 1
  spline S102 degree 2 poles (-2.7358, 19.816) (-2.5473, 20.1228) (-2.6394, 20.6712) knots 0 0 0 1 1 1
  spline S103 degree 2 poles (-2.6394, 20.6712) (-2.7261, 21.188) (-3.0057, 21.4149) knots 0 0 0 1 1 1
  spline S104 degree 2 poles (-3.0057, 21.4149) (-3.2852, 21.6417) (-3.6341, 21.5831) knots 0 0 0 1 1 1
  spline S105 degree 2 poles (-3.6341, 21.5831) (-3.9883, 21.5236) (-4.1773, 21.2194) knots 0 0 0 1 1 1
  spline S106 degree 2 poles (-4.1773, 21.2194) (-4.3663, 20.9152) (-4.2764, 20.38) knots 0 0 0 1 1 1
  line L47 (-1.3527, 19.3815) -> (-1.3814, 22.2066)
  line L48 (-1.3814, 22.2066) -> (-0.9505, 22.211)
  line L49 (-0.9505, 22.211) -> (-0.9464, 21.8093)
  spline S107 degree 2 poles (-0.9464, 21.8093) (-0.6399, 22.278) (-0.052, 22.2839) knots 0 0 0 1 1 1
  spline S108 degree 2 poles (-0.052, 22.2839) (0.2034, 22.2865) (0.4185, 22.1969) knots 0 0 0 1 1 1
  spline S109 degree 2 poles (0.4185, 22.1969) (0.6335, 22.1073) (0.7415, 21.9594) knots 0 0 0 1 1 1
  spline S110 degree 2 poles (0.7415, 21.9594) (0.8494, 21.8115) (0.894, 21.6071) knots 0 0 0 1 1 1
  spline S111 degree 2 poles (0.894, 21.6071) (0.922, 21.4744) (0.9253, 21.1419) knots 0 0 0 1 1 1
  line L50 (0.9253, 21.1419) -> (0.943, 19.4048)
  line L51 (0.943, 19.4048) -> (0.4642, 19.3999)
  line L52 (0.4642, 19.3999) -> (0.4467, 21.1184)
  spline S112 degree 2 poles (0.4467, 21.1184) (0.4437, 21.411) (0.3864, 21.5554) knots 0 0 0 1 1 1
  spline S113 degree 2 poles (0.3864, 21.5554) (0.3291, 21.6998) (0.1859, 21.7849) knots 0 0 0 1 1 1
  spline S114 degree 2 poles (0.1859, 21.7849) (0.0427, 21.8699) (-0.1489, 21.8679) knots 0 0 0 1 1 1
  spline S115 degree 2 poles (-0.1489, 21.8679) (-0.4548, 21.8648) (-0.6749, 21.6684) knots 0 0 0 1 1 1
  spline S116 degree 2 poles (-0.6749, 21.6684) (-0.8951, 21.4719) (-0.8896, 20.9293) knots 0 0 0 1 1 1
  line L53 (-0.8896, 20.9293) -> (-0.8739, 19.3864)
  line L54 (-0.8739, 19.3864) -> (-1.3527, 19.3815)
  line L55 (3.6142, 19.0679) -> (3.181, 19.1666)
  line L56 (3.181, 19.1666) -> (4.0478, 22.9691)
  line L57 (4.0478, 22.9691) -> (4.5147, 22.8626)
  line L58 (4.5147, 22.8626) -> (4.2055, 21.5061)
  spline S117 degree 2 poles (4.2055, 21.5061) (4.5857, 21.8096) (5.0448, 21.705) knots 0 0 0 1 1 1
  spline S118 degree 2 poles (5.0448, 21.705) (5.299, 21.647) (5.5026, 21.4928) knots 0 0 0 1 1 1
  spline S119 degree 2 poles (5.5026, 21.4928) (5.7062, 21.3386) (5.8105, 21.1198) knots 0 0 0 1 1 1
  spline S120 degree 2 poles (5.8105, 21.1198) (5.9147, 20.9009) (5.938, 20.62) knots 0 0 0 1 1 1
  spline S121 degree 2 poles (5.938, 20.62) (5.9613, 20.3391) (5.8933, 20.0408) knots 0 0 0 1 1 1
  spline S122 degree 2 poles (5.8933, 20.0408) (5.7319, 19.3327) (5.2936, 19.0261) knots 0 0 0 1 1 1
  spline S123 degree 2 poles (5.2936, 19.0261) (4.8554, 18.7195) (4.3651, 18.8312) knots 0 0 0 1 1 1
  spline S124 degree 2 poles (4.3651, 18.8312) (3.8775, 18.9424) (3.6928, 19.4129) knots 0 0 0 1 1 1
  line L59 (3.6928, 19.4129) -> (3.6142, 19.0679)
  spline S125 degree 2 poles (3.9277, 20.4671) (3.8147, 19.9717) (3.8994, 19.7205) knots 0 0 0 1 1 1
  spline S126 degree 2 poles (3.8994, 19.7205) (4.0376, 19.3097) (4.4137, 19.224) knots 0 0 0 1 1 1
  spline S127 degree 2 poles (4.4137, 19.224) (4.7198, 19.1542) (5.0035, 19.3692) knots 0 0 0 1 1 1
  spline S128 degree 2 poles (5.0035, 19.3692) (5.2871, 19.5842) (5.4072, 20.1107) knots 0 0 0 1 1 1
  spline S129 degree 2 poles (5.4072, 20.1107) (5.5302, 20.6502) (5.3747, 20.9558) knots 0 0 0 1 1 1
  spline S130 degree 2 poles (5.3747, 20.9558) (5.2193, 21.2614) (4.9158, 21.3305) knots 0 0 0 1 1 1
  spline S131 degree 2 poles (4.9158, 21.3305) (4.6097, 21.4003) (4.3261, 21.1853) knots 0 0 0 1 1 1
  spline S132 degree 2 poles (4.3261, 21.1853) (4.0424, 20.9703) (3.9277, 20.4671) knots 0 0 0 1 1 1
  spline S133 degree 2 poles (6.486, 19.8151) (6.7774, 20.5437) (7.3228, 20.7325) knots 0 0 0 1 1 1
  spline S134 degree 2 poles (7.3228, 20.7325) (7.7777, 20.8887) (8.2643, 20.6941) knots 0 0 0 1 1 1
  spline S135 degree 2 poles (8.2643, 20.6941) (8.8053, 20.4778) (9.0069, 19.9861) knots 0 0 0 1 1 1
  spline S136 degree 2 poles (9.0069, 19.9861) (9.2085, 19.4943) (8.9587, 18.8694) knots 0 0 0 1 1 1
  spline S137 degree 2 poles (8.9587, 18.8694) (8.7562, 18.363) (8.4882, 18.1335) knots 0 0 0 1 1 1
  spline S138 degree 2 poles (8.4882, 18.1335) (8.2203, 17.904) (7.8658, 17.8595) knots 0 0 0 1 1 1
  spline S139 degree 2 poles (7.8658, 17.8595) (7.5114, 17.815) (7.168, 17.9522) knots 0 0 0 1 1 1
  spline S140 degree 2 poles (7.168, 17.9522) (6.6172, 18.1725) (6.4188, 18.6615) knots 0 0 0 1 1 1
  spline S141 degree 2 poles (6.4188, 18.6615) (6.2204, 19.1506) (6.486, 19.8151) knots 0 0 0 1 1 1
  spline S142 degree 2 poles (6.943, 19.6323) (6.7415, 19.1284) (6.8611, 18.7898) knots 0 0 0 1 1 1
  spline S143 degree 2 poles (6.8611, 18.7898) (6.9807, 18.4512) (7.3142, 18.3178) knots 0 0 0 1 1 1
  spline S144 degree 2 poles (7.3142, 18.3178) (7.6452, 18.1855) (7.9658, 18.3495) knots 0 0 0 1 1 1
  spline S145 degree 2 poles (7.9658, 18.3495) (8.2864, 18.5136) (8.4928, 19.0299) knots 0 0 0 1 1 1
  spline S146 degree 2 poles (8.4928, 19.0299) (8.6874, 19.5165) (8.5665, 19.8556) knots 0 0 0 1 1 1
  spline S147 degree 2 poles (8.5665, 19.8556) (8.4457, 20.1947) (8.1172, 20.3261) knots 0 0 0 1 1 1
  spline S148 degree 2 poles (8.1172, 20.3261) (7.7837, 20.4594) (7.4641, 20.2978) knots 0 0 0 1 1 1
  spline S149 degree 2 poles (7.4641, 20.2978) (7.1445, 20.1362) (6.943, 19.6323) knots 0 0 0 1 1 1
  spline S150 degree 2 poles (10.6839, 16.6163) (10.3397, 16.558) (10.0806, 16.6037) knots 0 0 0 1 1 1
  spline S151 degree 2 poles (10.0806, 16.6037) (9.8215, 16.6495) (9.5792, 16.7937) knots 0 0 0 1 1 1
  spline S152 degree 2 poles (9.5792, 16.7937) (9.179, 17.0317) (9.0804, 17.355) knots 0 0 0 1 1 1
  spline S153 degree 2 poles (9.0804, 17.355) (8.9818, 17.6783) (9.1626, 17.9824) knots 0 0 0 1 1 1
  spline S154 degree 2 poles (9.1626, 17.9824) (9.2687, 18.1608) (9.4376, 18.26) knots 0 0 0 1 1 1
  spline S155 degree 2 poles (9.4376, 18.26) (9.6065, 18.3591) (9.791, 18.3701) knots 0 0 0 1 1 1
  spline S156 degree 2 poles (9.791, 18.3701) (9.9755, 18.3811) (10.1673, 18.3289) knots 0 0 0 1 1 1
  spline S157 degree 2 poles (10.1673, 18.3289) (10.3076, 18.2888) (10.5699, 18.173) knots 0 0 0 1 1 1
  spline S158 degree 2 poles (10.5699, 18.173) (11.1037, 17.936) (11.3881, 17.8782) knots 0 0 0 1 1 1
  spline S159 degree 2 poles (11.3881, 17.8782) (11.4407, 17.9615) (11.4543, 17.9843) knots 0 0 0 1 1 1
  spline S160 degree 2 poles (11.4543, 17.9843) (11.6039, 18.2358) (11.5485, 18.4081) knots 0 0 0 1 1 1
  spline S161 degree 2 poles (11.5485, 18.4081) (11.4737, 18.6414) (11.1628, 18.8263) knots 0 0 0 1 1 1
  spline S162 degree 2 poles (11.1628, 18.8263) (10.8724, 18.9991) (10.6736, 18.9796) knots 0 0 0 1 1 1
  spline S163 degree 2 poles (10.6736, 18.9796) (10.4747, 18.9601) (10.2547, 18.7412) knots 0 0 0 1 1 1
  line L60 (10.2547, 18.7412) -> (9.885, 19.0354)
  spline S164 degree 2 poles (9.885, 19.0354) (10.0935, 19.2612) (10.3138, 19.3453) knots 0 0 0 1 1 1
  spline S165 degree 2 poles (10.3138, 19.3453) (10.5341, 19.4294) (10.8228, 19.3737) knots 0 0 0 1 1 1
  spline S166 degree 2 poles (10.8228, 19.3737) (11.1116, 19.318) (11.4249, 19.1317) knots 0 0 0 1 1 1
  spline S167 degree 2 poles (11.4249, 19.1317) (11.7358, 18.9467) (11.8866, 18.7579) knots 0 0 0 1 1 1
  spline S168 degree 2 poles (11.8866, 18.7579) (12.0375, 18.5692) (12.063, 18.4039) knots 0 0 0 1 1 1
  spline S169 degree 2 poles (12.063, 18.4039) (12.0885, 18.2386) (12.0244, 18.0476) knots 0 0 0 1 1 1
  spline S170 degree 2 poles (12.0244, 18.0476) (11.9824, 17.9302) (11.8192, 17.6558) knots 0 0 0 1 1 1
  line L61 (11.8192, 17.6558) -> (11.4928, 17.1071)
  spline S171 degree 2 poles (11.4928, 17.1071) (11.1515, 16.5332) (11.0873, 16.3655) knots 0 0 0 1 1 1
  spline S172 degree 2 poles (11.0873, 16.3655) (11.0232, 16.1979) (11.0179, 16.0121) knots 0 0 0 1 1 1
  line L62 (11.0179, 16.0121) -> (10.5881, 16.2678)
  spline S173 degree 2 poles (10.5881, 16.2678) (10.6002, 16.4339) (10.6839, 16.6163) knots 0 0 0 1 1 1
  spline S174 degree 2 poles (11.1964, 17.5558) (10.9179, 17.5977) (10.4317, 17.8002) knots 0 0 0 1 1 1
  spline S175 degree 2 poles (10.4317, 17.8002) (10.1561, 17.9146) (10.0238, 17.9314) knots 0 0 0 1 1 1
  spline S176 degree 2 poles (10.0238, 17.9314) (9.8914, 17.9482) (9.7819, 17.8942) knots 0 0 0 1 1 1
  spline S177 degree 2 poles (9.7819, 17.8942) (9.6724, 17.8402) (9.6084, 17.7327) knots 0 0 0 1 1 1
  spline S178 degree 2 poles (9.6084, 17.7327) (9.5105, 17.5681) (9.5698, 17.3842) knots 0 0 0 1 1 1
  spline S179 degree 2 poles (9.5698, 17.3842) (9.6292, 17.2004) (9.8692, 17.0576) knots 0 0 0 1 1 1
  spline S180 degree 2 poles (9.8692, 17.0576) (10.107, 16.9161) (10.3541, 16.91) knots 0 0 0 1 1 1
  spline S181 degree 2 poles (10.3541, 16.91) (10.6012, 16.9039) (10.7955, 17.0328) knots 0 0 0 1 1 1
  spline S182 degree 2 poles (10.7955, 17.0328) (10.9448, 17.1329) (11.1066, 17.4049) knots 0 0 0 1 1 1
  line L63 (11.1066, 17.4049) -> (11.1964, 17.5558)
  line L64 (11.4779, 15.6442) -> (13.2177, 17.8702)
  line L65 (13.2177, 17.8702) -> (13.5573, 17.6048)
  line L66 (13.5573, 17.6048) -> (13.2935, 17.2674)
  spline S183 degree 2 poles (13.2935, 17.2674) (13.6086, 17.4026) (13.7776, 17.3921) knots 0 0 0 1 1 1
  spline S184 degree 2 poles (13.7776, 17.3921) (13.9467, 17.3815) (14.0787, 17.2783) knots 0 0 0 1 1 1
  spline S185 degree 2 poles (14.0787, 17.2783) (14.2694, 17.1292) (14.3715, 16.8537) knots 0 0 0 1 1 1
  line L67 (14.3715, 16.8537) -> (13.9679, 16.6052)
  spline S186 degree 2 poles (13.9679, 16.6052) (13.8935, 16.7951) (13.7551, 16.9032) knots 0 0 0 1 1 1
  spline S187 degree 2 poles (13.7551, 16.9032) (13.6315, 16.9999) (13.4748, 17.0025) knots 0 0 0 1 1 1
  spline S188 degree 2 poles (13.4748, 17.0025) (13.3181, 17.005) (13.173, 16.9058) knots 0 0 0 1 1 1
  spline S189 degree 2 poles (13.173, 16.9058) (12.9528, 16.7537) (12.7661, 16.5147) knots 0 0 0 1 1 1
  line L68 (12.7661, 16.5147) -> (11.8552, 15.3494)
  line L69 (11.8552, 15.3494) -> (11.4779, 15.6442)
  line L70 (14.2564, 13.1663) -> (14.5096, 13.4171)
  spline S190 degree 2 poles (14.5096, 13.4171) (14.0219, 13.3123) (13.655, 13.6827) knots 0 0 0 1 1 1
  spline S191 degree 2 poles (13.655, 13.6827) (13.4173, 13.9228) (13.3502, 14.2551) knots 0 0 0 1 1 1
  spline S192 degree 2 poles (13.3502, 14.2551) (13.2831, 14.5875) (13.4109, 14.933) knots 0 0 0 1 1 1
  spline S193 degree 2 poles (13.4109, 14.933) (13.5386, 15.2785) (13.8467, 15.5836) knots 0 0 0 1 1 1
  spline S194 degree 2 poles (13.8467, 15.5836) (14.1472, 15.8813) (14.4912, 16.0235) knots 0 0 0 1 1 1
  spline S195 degree 2 poles (14.4912, 16.0235) (14.8352, 16.1658) (15.164, 16.0946) knots 0 0 0 1 1 1
  spline S196 degree 2 poles (15.164, 16.0946) (15.4929, 16.0234) (15.7381, 15.7758) knots 0 0 0 1 1 1
  spline S197 degree 2 poles (15.7381, 15.7758) (15.9178, 15.5943) (15.9817, 15.3767) knots 0 0 0 1 1 1
  spline S198 degree 2 poles (15.9817, 15.3767) (16.0455, 15.1592) (16.0107, 14.9486) knots 0 0 0 1 1 1
  line L71 (16.0107, 14.9486) -> (17.0049, 15.9333)
  line L72 (17.0049, 15.9333) -> (17.34, 15.595)
  line L73 (17.34, 15.595) -> (14.569, 12.8506)
  line L74 (14.569, 12.8506) -> (14.2564, 13.1663)
  spline S199 degree 2 poles (14.193, 15.234) (13.8074, 14.8521) (13.7775, 14.5004) knots 0 0 0 1 1 1
  spline S200 degree 2 poles (13.7775, 14.5004) (13.7475, 14.1488) (13.9666, 13.9277) knots 0 0 0 1 1 1
  spline S201 degree 2 poles (13.9666, 13.9277) (14.1875, 13.7046) (14.5243, 13.7293) knots 0 0 0 1 1 1
  spline S202 degree 2 poles (14.5243, 13.7293) (14.8612, 13.754) (15.2354, 14.1247) knots 0 0 0 1 1 1
  spline S203 degree 2 poles (15.2354, 14.1247) (15.6475, 14.5328) (15.683, 14.8825) knots 0 0 0 1 1 1
  spline S204 degree 2 poles (15.683, 14.8825) (15.7186, 15.2322) (15.4883, 15.4647) knots 0 0 0 1 1 1
  spline S205 degree 2 poles (15.4883, 15.4647) (15.2637, 15.6915) (14.9277, 15.6602) knots 0 0 0 1 1 1
  spline S206 degree 2 poles (14.9277, 15.6602) (14.5918, 15.629) (14.193, 15.234) knots 0 0 0 1 1 1
  spline S207 degree 2 poles (17.0856, 11.9494) (17.7562, 12.3571) (18.3056, 12.1805) knots 0 0 0 1 1 1
  spline S208 degree 2 poles (18.3056, 12.1805) (18.7632, 12.0322) (19.0355, 11.5844) knots 0 0 0 1 1 1
  spline S209 degree 2 poles (19.0355, 11.5844) (19.3381, 11.0866) (19.204, 10.5723) knots 0 0 0 1 1 1
  spline S210 degree 2 poles (19.204, 10.5723) (19.0699, 10.058) (18.4948, 9.7083) knots 0 0 0 1 1 1
  spline S211 degree 2 poles (18.4948, 9.7083) (18.0289, 9.425) (17.6768, 9.4024) knots 0 0 0 1 1 1
  spline S212 degree 2 poles (17.6768, 9.4024) (17.3247, 9.3798) (17.0145, 9.5571) knots 0 0 0 1 1 1
  spline S213 degree 2 poles (17.0145, 9.5571) (16.7044, 9.7343) (16.5123, 10.0503) knots 0 0 0 1 1 1
  spline S214 degree 2 poles (16.5123, 10.0503) (16.2041, 10.5572) (16.3391, 11.0674) knots 0 0 0 1 1 1
  spline S215 degree 2 poles (16.3391, 11.0674) (16.4741, 11.5776) (17.0856, 11.9494) knots 0 0 0 1 1 1
  spline S216 degree 2 poles (17.3413, 11.5288) (16.8776, 11.2469) (16.7698, 10.9043) knots 0 0 0 1 1 1
  spline S217 degree 2 poles (16.7698, 10.9043) (16.6621, 10.5617) (16.8487, 10.2548) knots 0 0 0 1 1 1
  spline S218 degree 2 poles (16.8487, 10.2548) (17.0339, 9.9502) (17.3888, 9.8889) knots 0 0 0 1 1 1
  spline S219 degree 2 poles (17.3888, 9.8889) (17.7436, 9.8276) (18.2187, 10.1164) knots 0 0 0 1 1 1
  spline S220 degree 2 poles (18.2187, 10.1164) (18.6665, 10.3887) (18.7735, 10.7324) knots 0 0 0 1 1 1
  spline S221 degree 2 poles (18.7735, 10.7324) (18.8806, 11.0761) (18.6968, 11.3784) knots 0 0 0 1 1 1
  spline S222 degree 2 poles (18.6968, 11.3784) (18.5102, 11.6853) (18.1576, 11.748) knots 0 0 0 1 1 1
  spline S223 degree 2 poles (18.1576, 11.748) (17.805, 11.8108) (17.3413, 11.5288) knots 0 0 0 1 1 1
  line L75 (17.5193, 8.3279) -> (19.7546, 9.3376)
  line L76 (19.7546, 9.3376) -> (19.5805, 9.7231)
  line L77 (19.5805, 9.7231) -> (19.9199, 9.8764)
  line L78 (19.9199, 9.8764) -> (20.094, 9.491)
  line L79 (20.094, 9.491) -> (20.368, 9.6147)
  spline S224 degree 2 poles (20.368, 9.6147) (20.6274, 9.7319) (20.7743, 9.7428) knots 0 0 0 1 1 1
  spline S225 degree 2 poles (20.7743, 9.7428) (20.9725, 9.7564) (21.1496, 9.6452) knots 0 0 0 1 1 1
  spline S226 degree 2 poles (21.1496, 9.6452) (21.3268, 9.5341) (21.4561, 9.248) knots 0 0 0 1 1 1
  spline S227 degree 2 poles (21.4561, 9.248) (21.5393, 9.0637) (21.5964, 8.821) knots 0 0 0 1 1 1
  line L80 (21.5964, 8.821) -> (21.1862, 8.7145)
  spline S228 degree 2 poles (21.1862, 8.7145) (21.1491, 8.8612) (21.0944, 8.9824) knots 0 0 0 1 1 1
  spline S229 degree 2 poles (21.0944, 8.9824) (21.0046, 9.1812) (20.8825, 9.2253) knots 0 0 0 1 1 1
  spline S230 degree 2 poles (20.8825, 9.2253) (20.7604, 9.2694) (20.5276, 9.1643) knots 0 0 0 1 1 1
  line L81 (20.5276, 9.1643) -> (20.29, 9.057)
  line L82 (20.29, 9.057) -> (20.5167, 8.5551)
  line L83 (20.5167, 8.5551) -> (20.1773, 8.4018)
  line L84 (20.1773, 8.4018) -> (19.9506, 8.9037)
  line L85 (19.9506, 8.9037) -> (17.7153, 7.894)
  line L86 (17.7153, 7.894) -> (17.5193, 8.3279)
  line L87 (19.308, 4.5337) -> (18.9176, 4.3568)
  spline S231 degree 2 poles (18.9176, 4.3568) (18.8239, 4.5409) (18.7823, 4.695) knots 0 0 0 1 1 1
  spline S232 degree 2 poles (18.7823, 4.695) (18.7145, 4.9468) (18.7567, 5.1069) knots 0 0 0 1 1 1
  spline S233 degree 2 poles (18.7567, 5.1069) (18.7989, 5.2671) (18.9134, 5.3586) knots 0 0 0 1 1 1
  spline S234 degree 2 poles (18.9134, 5.3586) (19.0279, 5.4501) (19.444, 5.5622) knots 0 0 0 1 1 1
  line L88 (19.444, 5.5622) -> (21.0135, 5.9853)
  line L89 (21.0135, 5.9853) -> (20.9221, 6.3243)
  line L90 (20.9221, 6.3243) -> (21.2817, 6.4213)